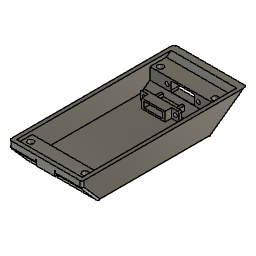
v2 - Timer - Battery box (Autodesk Fusion 360 design; units mm, degrees)
Autodesk Fusion 360 part; units mm, degrees
note: some values were not read from the file. Set by a fixed rule: which sketch regions a step uses.
sketch "Box side" plane through (0, 0, 0) normal (1, 0, 0) x (0, 1, 0)
  line L0 (127, 20) -> (0, 20)
  line L1 (0, 20) -> (0, 15)
  line L2 (0, 15) -> (13.228757, 0)
  line L3 (127, 20) -> (99.228757, 0)
  line L4 (13.228757, 0) -> (99.228757, 0)
  dimension "d2" = 20
  dimension "d3" = 5
  dimension "d4" = 86
  dimension "d5" = 20
  dimension "d6" = 127
  constraint horizontal L0
  measures "d2" distance of origin L0.end
  measures "d3" distance of L0.end L1.end
  measures "d6" distance of L0.start L0.end
extrude "Extrude1" add sketch "Box side" along normal blind 56 contours L0 L1 L2 L3 L4 picked at (75.409586, 13.333333) makes body 1
shell "Shell1" thickness 3 removed faces 1 at (37.333333, 84.666667, 20) on bodies 1
fillet "Fillet1" radius 1.5 1 edges at (56, 6.614378, 7.5) on bodies 1
fillet "Fillet2" radius 1.5 2 edges at (56, 113.114378, 10) (0, 113.114378, 10) on bodies 1
fillet "Fillet3" radius 1.5 1 edges at (0, 6.614378, 7.5) on bodies 1
fillet "Fillet4" radius 1.5 5 edges at (0, 0, 18.633893) (0.43934, 0, 15.664219) (28, 0, 15) (55.56066, 0, 15.664219) (56, 0, 18.633893) on bodies 1
fillet "Fillet5" radius 1.5 8 edges at (56, 55.945379, 0) (55.56066, 98.476971, 0) (28, 99.228757, 0) (0.43934, 98.476971, 0) (0, 55.945379, 0) (0.43934, 13.814543, 0) (28, 13.228757, 0) (55.56066, 13.814543, 0) on bodies 1
sketch "Holes" plane through (0, 0, 20) normal (0, 0, 1) x (-1, 0, 0)
  arc A0 (-54.5, 0) -> (-56, -1.5) centre (-54.5, -1.5) ccw
  line L0 (-56, -1.5) -> (-56, -124.433244)
  ellipse E0 centre (-54.5, -124.433244) end of major axis (-54.5, -127) minor radius 1.5 (-56, -124.433244) -> (-54.5, -127) ccw
  line L1 (-54.5, -127) -> (-1.5, -127)
  ellipse E1 centre (-1.5, -124.433244) end of major axis (-1.5, -127) minor radius 1.5 (-1.5, -127) -> (0, -124.433244) ccw
  line L2 (0, -124.433244) -> (0, -1.5)
  arc A1 (0, -1.5) -> (-1.5, 0) centre (-1.5, -1.5) ccw
  line L3 (-1.5, 0) -> (-54.5, 0)
  line L4 (-53, -3) -> (-3, -3)
  line L5 (-3, -3) -> (-3, -121.866488)
  line L6 (-3, -121.866488) -> (-53, -121.866488)
  line L7 (-53, -121.866488) -> (-53, -3)
  line L8 (0, 0) -> (-56, 0)
  line L9 (-56, 0) -> (-56, -127)
  line L10 (-56, -127) -> (0, -127)
  line L11 (0, -127) -> (0, 0)
  circle A2 centre (-7, -9.59) radius 2.3
  line L12 (0, -127) -> (0, 0)
  circle A3 centre (-49, -9.59) radius 2.3
  circle A4 centre (-7, -109.59) radius 2.3
  circle A5 centre (-49, -109.59) radius 2.3
  line L13 (0, 0) -> (-56, 0)
  line L14 (-56, 0) -> (-56, -15)
  line L15 (-56, -15) -> (0, -15)
  line L16 (0, -15) -> (0, 0)
  line L17 (-11, -105.59) -> (-3, -105.59)
  line L18 (-3, -105.59) -> (-3, -113.59)
  line L19 (-3, -113.59) -> (-11, -113.59)
  line L20 (-11, -113.59) -> (-11, -105.59)
  line L21 (-11, -105.59) -> (-3, -113.59) construction
  line L22 (-3, -105.59) -> (-11, -113.59) construction
  line L23 (-53, -105.59) -> (-45, -105.59)
  line L24 (-45, -105.59) -> (-45, -113.59)
  line L25 (-45, -113.59) -> (-53, -113.59)
  line L26 (-53, -113.59) -> (-53, -105.59)
  line L27 (-53, -105.59) -> (-45, -113.59) construction
  line L28 (-45, -105.59) -> (-53, -113.59) construction
  point P0 (-7, -109.59)
  point P1 (-49, -109.59)
  dimension "d25" = 56
  dimension "d26" = 4.6
  dimension "d27" = 9.59
  dimension "d28" = 7
  dimension "d29" = 4.6
  dimension "d30" = 7
  dimension "d31" = 9.59
  dimension "d32" = 4.6
  dimension "d33" = 17.41
  dimension "d34" = 7
  dimension "d35" = 4.6
  dimension "d36" = 7
  dimension "d37" = 17.41
  dimension "d38" = 15
  dimension "d47" = 8
  dimension "d48" = 8
  dimension "d49" = 8
  dimension "d50" = 8
  constraint horizontal L8
  constraint vertical L9
  constraint horizontal L10
  constraint vertical L11
  constraint coincident L8.start L11.end
  constraint horizontal L13
  constraint vertical L14
  constraint horizontal L15
  constraint vertical L16
  constraint horizontal L17
  constraint perpendicular L17 L18
  constraint parallel L17 L19
  constraint parallel L18 L20
  constraint coincident L21 P0
  constraint coincident L22 P0
  constraint coincident P0 A4.centre
  constraint horizontal L23
  constraint perpendicular L23 L24
  constraint parallel L23 L25
  constraint parallel L24 L26
  constraint coincident L27 P1
  constraint coincident L28 P1
  constraint coincident P1 A5.centre
  measures "d25" distance of L8.start L8.end
  measures "d26" diameter of A2
  measures "d27" distance of L8 A2.centre
  measures "d28" distance of A2.centre L12
  measures "d29" diameter of A3
  measures "d30" distance of L9 A3.centre
  measures "d31" distance of L8 A3.centre
  measures "d32" diameter of A4
  measures "d33" distance of L10 P0
  measures "d34" distance of L12 P0
  measures "d35" diameter of A5
  measures "d36" distance of L9 P1
  measures "d37" distance of L10 P1
  measures "d38" distance of L8.start L15.end
  measures "d47" distance of L18.end L19.end
  measures "d48" distance of L17.end L18.end
  measures "d49" distance of L24.end L25.end
  measures "d50" distance of L23.end L24.end
sketch "Sketch5" plane through (56, 0, 0) normal (1, 0, 0) x (0, 1, 0)
  line L0 (13.905881, 1.5) -> (98.744844, 1.5)
  line L1 (98.744844, 1.5) -> (124.433244, 20)
  line L2 (124.433244, 20) -> (1.5, 20)
  line L3 (1.5, 20) -> (1.5, 15.566947)
  line L4 (1.5, 15.566947) -> (13.905881, 1.5)
  line L5 (0, 0) -> (15, 0)
  line L6 (15, 0) -> (15, 20)
  line L7 (15, 20) -> (0, 20)
  line L8 (0, 20) -> (0, 0)
  line L9 (0, 20) -> (105.59, 20)
  line L10 (105.59, 20) -> (105.59, 0)
  line L11 (105.59, 0) -> (0, 0)
  line L12 (0, 0) -> (0, 20)
  line L13 (105.59, 20) -> (113.59, 20)
  line L14 (113.59, 20) -> (113.59, 0)
  line L15 (113.59, 0) -> (105.59, 0)
  line L16 (105.59, 0) -> (105.59, 20)
  dimension "d51" = 105.59
  dimension "d52" = 8
  constraint horizontal L5
  constraint vertical L6
  constraint horizontal L7
  constraint vertical L8
  constraint coincident L2 L6.end
  constraint coincident L5.start L8.end
  constraint horizontal L9
  constraint vertical L10
  constraint horizontal L11
  constraint vertical L12
  constraint horizontal L13
  constraint vertical L14
  constraint horizontal L15
  constraint vertical L16
  measures "d51" distance of L7.end L9.end
  measures "d52" distance of L9.end L13.end
extrude "Extrude2" add sketch "Sketch5" against normal blind 56 contours L0 L2 L3 L4 L6 L7 L9 picked at (10.135294, 12.355649) bodies 1
extrude "Extrude3" cut sketch "Holes" against normal blind 2.5 contours L4 L5 L7 L15 picked at (-34.521991, -4.597263) bodies 1
extrude "Extrude4" cut 2 faces at (6.942707, 11.397454, 20) (48.521991, 9.737446, 20) along direction (0, 0, -1) blind 9.5 on bodies 1 bodies 1
extrude "Extrude5" cut 1 faces at (34.521991, 4.597263, 17.5) along direction (0, 0, -1) blind 0.2 on bodies 1 bodies 1
extrude "Extrude6" add sketch "Sketch5" against normal blind 56 contours L1 L2 L10 L13 L14 L16 picked at (108.256667, 12.873566) bodies 1
extrude "Extrude7" cut sketch "Holes" against normal blind 2.7 contours L7 L23 L24 L25 L26 | L5 L17 L18 L19 L20 picked at (-49.057293, -113.02119) picked at (-6.942707, -113.02119) bodies 1
extrude "Extrude8" cut sketch "Holes" against normal blind 9.7 contours A4 | A5 picked at (-7.170599, -111.002733) picked at (-49.732606, -108.32109) bodies 1
extrude "Extrude9" cut 1 faces at (6.942707, 11.397454, 10.5) along direction (0, 0, -1) blind 0.2 on bodies 1 bodies 1
extrude "Extrude10" cut 1 faces at (48.521991, 9.737446, 10.5) along direction (0, 0, -1) blind 0.2 on bodies 1 bodies 1
extrude "Extrude11" cut 1 faces at (33.666667, 108.256667, 20) along direction (0, 0, -1) blind 2.7 on bodies 1 bodies 1
extrude "Extrude12" cut 1 faces at (53, 72.95031, 12.533333) along direction (1, 0, 0) blind 0.2 on bodies 1 bodies 1
extrude "Extrude13" cut 1 faces at (3, 72.95031, 12.533333) along direction (-1, 0, 0) blind 0.2 on bodies 1 bodies 1
extrude "Extrude14" add 1 faces at (21.478009, 4.597263, 17.3) along direction (0, 0, 1) blind 2.5 on bodies 1 bodies 1
sketch "Sketch7" plane through (0, 0, 0) normal (0, 1, 0) x (1, 0, 0)
  line L0 (0, -20) -> (56.000001, -20)
  line L1 (56.000001, -20) -> (56.000001, 0)
  line L2 (56.000001, 0) -> (0, 0)
  line L3 (0, 0) -> (0, -20)
  line L4 (35.5, -12) -> (20.5, -12)
  line L5 (20.5, -12) -> (20.5, -17)
  line L6 (20.5, -17) -> (35.5, -17)
  line L7 (35.5, -17) -> (35.5, -12)
  line L8 (35.5, -12) -> (20.5, -17) construction
  line L9 (20.5, -12) -> (35.5, -17) construction
  point P0 (28, -14.5)
  dimension "d75" = 56
  dimension "d76" = 20
  dimension "d77" = 15
  dimension "d79" = 5
  dimension "d80" = 28
  dimension "d83" = 3
  constraint horizontal L0
  constraint vertical L1
  constraint horizontal L2
  constraint vertical L3
  constraint horizontal L4
  constraint perpendicular L4 L5
  constraint parallel L4 L6
  constraint parallel L5 L7
  constraint coincident L8 P0
  constraint coincident L9 P0
  constraint coincident L2.end L3.start
  measures "d75" distance of L1 L3
  measures "d76" distance of L0 L2
  measures "d77" distance of L5 L7
  measures "d79" distance of L4 L6
  measures "d80" distance of L3 P0
  measures "d83" distance of L0 L6
extrude "Extrude16" cut sketch "Sketch7" along normal blind 5 contours L4 L5 L6 L7 picked at (25.5, -13.666667) bodies 1
sketch "Sketch9" plane through (0, 0, 17) normal (0, 0, -1) x (1, 0, 0)
  line L0 (35.5, 0) -> (20.5, 0)
  line L1 (20.5, 0) -> (20.5, -5)
  line L2 (20.5, -5) -> (35.5, -5)
  line L3 (35.5, -5) -> (35.5, 0)
  line L4 (21, 0) -> (35, 0)
  line L5 (35, 0) -> (35, -4)
  line L6 (35, -4) -> (21, -4)
  line L7 (21, -4) -> (21, 0)
  line L8 (21, 0) -> (35, -4) construction
  line L9 (35, 0) -> (21, -4) construction
  line L10 (0, -124.433244) -> (0, -1.5)
  point P0 (28, -2)
  dimension "d86" = 14
  dimension "d87" = 4
  dimension "d88" = 28
  constraint horizontal L4
  constraint perpendicular L4 L5
  constraint parallel L4 L6
  constraint parallel L5 L7
  constraint coincident L8 P0
  constraint coincident L9 P0
  measures "d86" distance of L5.end L6.end
  measures "d87" distance of L4.end L5.end
  measures "d88" distance of P0 L10
extrude "Extrude17" add sketch "Sketch9" along normal blind 4 contours L0 L4 L5 L6 L7 picked at (25.666667, -2.666667) bodies 1
sketch "Sketch10" plane through (0, 0, 0) normal (0, 0, -1) x (1, 0, 0)
  line L0 (54.5, -98.744844) -> (54.5, -13.905881)
  line L1 (54.5, -13.905881) -> (1.5, -13.905881)
  line L2 (1.5, -13.905881) -> (1.5, -98.744844)
  line L3 (1.5, -98.744844) -> (54.5, -98.744844)
  line L4 (0, 0) -> (56, 0)
  line L5 (56, 0) -> (56, -40)
  line L6 (56, -40) -> (0, -40)
  line L7 (0, -40) -> (0, 0)
  circle A0 centre (28, -23.905881) radius 7.5
  circle A1 centre (28, -23.905881) radius 8
  circle A2 centre (28, -23.905881) radius 7.5
  line L8 (28, -23.905881) -> (28, -16.405881)
  line L9 (28, -23.905881) -> (28, -31.405881)
  line L10 (26, -18) -> (23.547729, -27.718074)
  line L11 (30, -18) -> (32.224339, -27.773881)
  line L12 (26, -18) -> (28, -27.655881)
  line L13 (30, -18) -> (28, -27.655881)
  spline S0 degree 2 poles (23.547729, -27.718074) (25.851156, -26.785289) (28, -27.655881) knots 0 0 0 0.45428894 0.45428894 0.45428894
  spline S1 degree 2 poles (28, -27.655881) (29.871062, -26.736857) (32.224339, -27.773881) knots 0 0 0 0.43365023 0.43365023 0.43365023
  dimension "d91" = 56
  dimension "d92" = 40
  dimension "d93" = 15
  dimension "d94" = 28
  dimension "d95" = 10
  dimension "d96" = 16
  constraint horizontal L4
  constraint vertical L5
  constraint horizontal L6
  constraint vertical L7
  constraint coincident L4.start L7.end
  constraint concentric A0 A1
  constraint concentric A0 A2
  constraint vertical L8
  constraint parallel L8 L9
  measures "d91" distance of L4.start L4.end
  measures "d92" distance of L4.start L6.end
  measures "d93" diameter of A0
  measures "d96" diameter of A1
extrude "Extrude18" cut sketch "Sketch10" against normal blind 1 contours L11 L13 S1 | L10 L12 S0 | A1 picked at (30.498904, -24.211617) picked at (25.626227, -24.177575) picked at (23.228629, -17.92277) bodies 1
sketch "Sketch13" plane through (0, 0, 0) normal (0, 1, 0) x (1, 0, 0)
ref_plane "WorkPlane1" through (28, 0, 16.5) normal (0, -1, 0) x (0, 0, -1)
ref_plane "WorkPlane3" through (0, 90, 0) normal (0, 1, 0) x (0, 0, 1)
sketch "Sketch19" plane through (0, 90, 0) normal (0, 1, 0) x (1, 0, 0)
  line L0 (0, 0) -> (56, 0)
  line L1 (56, 0) -> (56, -20)
  line L2 (56, -20) -> (0, -20)
  line L3 (0, -20) -> (0, 0)
  line L4 (37, -8.5) -> (19, -8.5)
  line L5 (19, -8.5) -> (19, -16)
  line L6 (19, -16) -> (37, -16)
  line L7 (37, -16) -> (37, -8.5)
  line L8 (37, -8.5) -> (19, -16) construction
  line L9 (19, -8.5) -> (37, -16) construction
  line L10 (19, -16) -> (13, -16)
  line L11 (13, -16) -> (13, -8.5)
  line L12 (13, -8.5) -> (19, -8.5)
  line L13 (19, -8.5) -> (19, -16)
  line L14 (37, -16) -> (43, -16)
  line L15 (43, -16) -> (43, -8.5)
  line L16 (43, -8.5) -> (37, -8.5)
  line L17 (37, -8.5) -> (37, -16)
  circle A0 centre (16, -12.25) radius 1.5
  circle A1 centre (40, -12.25) radius 1.5
  point P0 (28, -12.25)
  dimension "d185" = 56
  dimension "d186" = 20
  dimension "d187" = 18
  dimension "d188" = 7.5
  dimension "d189" = 28
  dimension "d190" = 4
  dimension "d191" = 6
  dimension "d192" = 3
  dimension "d193" = 3
  dimension "d194" = 3
  dimension "d195" = 3.75
  dimension "d196" = 3
  dimension "d197" = 3.75
  constraint horizontal L0
  constraint vertical L1
  constraint horizontal L2
  constraint vertical L3
  constraint coincident L0.start L3.end
  constraint horizontal L4
  constraint perpendicular L4 L5
  constraint parallel L5 L7
  constraint coincident L8 P0
  constraint coincident L9 P0
  constraint horizontal L10
  constraint vertical L11
  constraint horizontal L12
  constraint vertical L13
  constraint horizontal L14
  constraint vertical L15
  constraint horizontal L16
  constraint vertical L17
  constraint equal L12 L16
  constraint equal L5 L11
  constraint equal L7 L15
  measures "d185" distance of L0.start L0.end
  measures "d186" distance of L0.start L2.end
  measures "d187" distance of L5.end L6.end
  measures "d188" distance of L4.end L5.end
  measures "d189" distance of L3 P0
  measures "d190" distance of L2 L6
  measures "d191" distance of L5 L11
  measures "d192" diameter of A0
  measures "d193" diameter of A1
  measures "d194" distance of L11 A0.centre
  measures "d195" distance of L12 A0.centre
  measures "d196" distance of L7 A1.centre
  measures "d197" distance of L14 A1.centre
extrude "Extrude39" cut sketch "Sketch19" along normal blind 46 contours L4 L5 L6 L7 L13 L17 picked at (25, -13.5) bodies 1
extrude "Extrude40" cut 1 faces at (10.933333, 113.59, 15.126351) along direction (0, 1, 0) blind 4 on bodies 1 bodies 1
extrude "Extrude41" add 1 faces at (10.933333, 113.59, 15.126351) along direction (0, 1, 0) blind 5 on bodies 1 bodies 1
fillet "Fillet8" radius 1 4 edges at (37, 113.517876, 16) (37, 108.310768, 8.5) (19, 108.310768, 8.5) (19, 113.517876, 16) on bodies 1
extrude "Extrude42" cut sketch "Sketch19" along normal blind 19 contours A0 | A1 picked at (16.263967, -12.922576) picked at (40.344312, -12.057291) bodies 1
extrude "Extrude62" add sketch "Sketch19" against normal blind 2 separate body contours L7 L14 L15 L16 L17 | L5 L10 L11 L12 L13 picked at (40.037365, -9.251398) picked at (15.962635, -15.248602) makes body 2 at (15.962635, 90, 15.248602) makes body 3 at (40.037365, 90, 9.251398)
extrude "Extrude63" add sketch "Sketch19" against normal blind 7 contours L4 L5 L6 L7 L13 L17 picked at (25, -13.5) bodies 2 3
extrude "Extrude64" add sketch "Sketch19" along normal blind 8 contours L4 L5 L6 L7 L13 L17 picked at (25, -13.5) bodies 2
sketch "Sketch23" plane through (0, 83, 0) normal (0, -1, 0) x (1, 0, 0)
  line L0 (19, 16) -> (19, 8.5)
  line L1 (19, 8.5) -> (37, 8.5)
  line L2 (37, 8.5) -> (37, 16)
  line L3 (37, 16) -> (19, 16)
  line L4 (35.2, 10.05) -> (20.8, 10.05)
  line L5 (20.8, 10.05) -> (20.8, 14.45)
  line L6 (20.8, 14.45) -> (35.2, 14.45)
  line L7 (35.2, 14.45) -> (35.2, 10.05)
  line L8 (35.2, 10.05) -> (20.8, 14.45) construction
  line L9 (20.8, 10.05) -> (35.2, 14.45) construction
  line L10 (43, 16) -> (43, 8.5)
  line L11 (19, 16) -> (37, 16)
  point P0 (28, 12.25)
  dimension "d259" = 14.4
  dimension "d260" = 4.4
  dimension "d261" = 15
  dimension "d262" = 3.75
  constraint horizontal L4
  constraint perpendicular L4 L5
  constraint parallel L4 L6
  constraint parallel L5 L7
  constraint coincident L8 P0
  constraint coincident L9 P0
  measures "d259" distance of L5.end L6.end
  measures "d260" distance of L4.end L5.end
  measures "d261" distance of P0 L10
  measures "d262" distance of P0 L11
extrude "Extrude65" cut sketch "Sketch23" against normal blind 30 contours L4 L5 L6 L7 picked at (25.6, 11.516667) bodies 2
sketch "Sketch24" plane through (0, 98, 0) normal (0, 1, 0) x (-1, 0, 0)
  line L0 (-20.8, 14.45) -> (-20.8, 10.05)
  line L1 (-20.8, 10.05) -> (-35.2, 10.05)
  line L2 (-35.2, 10.05) -> (-35.2, 14.45)
  line L3 (-35.2, 14.45) -> (-20.8, 14.45)
  line L4 (-19, 8.5) -> (-19, 16)
  line L5 (-19, 16) -> (-37, 16)
  line L6 (-37, 16) -> (-37, 8.5)
  line L7 (-37, 8.5) -> (-19, 8.5)
  line L8 (-37, 8.5) -> (-19, 8.5)
  line L9 (-19, 8.5) -> (-19, 12.25)
  line L10 (-19, 12.25) -> (-37, 12.25)
  line L11 (-37, 12.25) -> (-37, 8.5)
  constraint horizontal L8
  constraint vertical L9
  constraint horizontal L10
  constraint vertical L11
  constraint midpoint L4 L9.end
  constraint coincident L6.end L7.start
extrude "Extrude66" cut sketch "Sketch24" against normal blind 8 contours L0 L2 L3 L4 L5 L6 L10 picked at (-30.4, 15.483333) bodies 2
sketch "Sketch25" plane through (0, 0, 10.05) normal (0, 0, 1) x (-1, 0, 0)
  line L0 (-35.2, -98) -> (-20.8, -98)
  line L1 (-20.8, -98) -> (-20.8, -83)
  line L2 (-20.8, -83) -> (-35.2, -83)
  line L3 (-35.2, -83) -> (-35.2, -98)
  circle A0 centre (-33.2, -92) radius 1.4
  circle A1 centre (-22.8, -92) radius 1.4
  dimension "d267" = 2.8
  dimension "d268" = 2.8
  dimension "d269" = 9
  dimension "d270" = 9
  dimension "d271" = 2
  dimension "d272" = 2
  measures "d267" diameter of A0
  measures "d268" diameter of A1
  measures "d269" distance of L2 A0.centre
  measures "d270" distance of L2 A1.centre
  measures "d271" distance of L1 A1.centre
  measures "d272" distance of L3 A0.centre
extrude "Extrude68" cut 1 faces at (31, 86.333333, 16) along direction (0, 0, -1) blind 0.2 on bodies 2 bodies 2
extrude "Extrude69" cut 1 faces at (43, 89.333333, 13.366667) along direction (-1, 0, 0) blind 0.2 on bodies 2 bodies 2
extrude "Extrude70" cut 1 faces at (13, 89.333333, 13.366667) along direction (1, 0, 0) blind 0.2 on bodies 2 bodies 2
extrude "Extrude71" cut 1 faces at (25, 95.333333, 8.5) along direction (0, 0, 1) blind 0.2 on bodies 2 bodies 2
fillet "Fillet10" radius 1 2 edges at (42.8, 89, 15.8) (13.2, 89, 15.8) on bodies 2
fillet "Fillet11" radius 1 2 edges at (42.8, 89, 8.7) (13.2, 89, 8.7) on bodies 2
extrude "Extrude72" cut sketch "Sketch25" against normal blind 3 contours A0 | A1 picked at (-33.096157, -92.454966) picked at (-23.526563, -91.737117) bodies 2
extrude "Extrude73" cut 1 faces at (21.478009, 4.597263, 19.8) along direction (0, 0, -1) blind 2.5 on bodies 1 bodies 1
equation "d194 = d191 / 2"
equation "d195 = d188 / 2"
equation "d196 = d191 / 2"
equation "d197 = d188 / 2"
equation "d262 = ( 7.5 / 2 ) * 1 mm"
